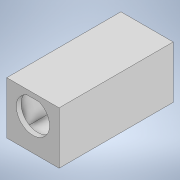
# Autodesk Inventor part: carcasaXeotype_FLEX-SENSOR
Saved by Autodesk Inventor 2020 (Build 240168000, 168)
## iProperties
Created: 2021-04-10
Part Number: carcasaXeotype_FLEX-SENSOR
Material: Generic
Document SubType Name: Modeling
Designer: Vlasciar
Density: 1 g/cm^3
Appearance: Default
Author: Vlasciar
Autodesk Inventor part; units mm, degrees
ref_plane "YZ Plane" through (0, 0, 0) normal (1, 0, 0) x (0, 1, 0)
ref_plane "XZ Plane" through (0, 0, 0) normal (0, 1, 0) x (-1, 0, 0)
ref_plane "XY Plane" through (0, 0, 0) normal (0, 0, 1) x (1, 0, 0)
sketch "Sketch1" plane through (0, 0, 0) normal (0, 1, 0) x (-1, 0, 0)
  line L0 (-5.5, -12) -> (5.5, -12)
  line L1 (5.5, -12) -> (5.5, 12)
  line L2 (5.5, 12) -> (-5.5, 12)
  line L3 (-5.5, 12) -> (-5.5, -12)
  line L4 (-5.5, -12) -> (5.5, 12) construction
  line L5 (5.5, -12) -> (-5.5, 12) construction
  point P0 (0, 0)
  dimension "d0" = 11
  dimension "d1" = 24
  constraints: 12 end point, 2 midpoint, 2 parallel, 1 horizontal, 1 perpendicular
  measures "d0" distance of L1.end L2.end
  measures "d1" distance of L0.end L1.end
extrude "Extrusion1" add sketch "Sketch1" along normal blind 10
shell "Shell1" thickness 1 removed faces 1 at (1.8333, 10, 4)
sketch "Sketch2" plane through (-5.5, 0, 12) normal (0, 0, 1) x (1, 0, 0)
  line L0 (0, 10) -> (11, 10) projected
  circle A0 centre (5.5, 6.75) radius 3.5
  point P0 (5.5, 0)
  point P1 (4.201, 10)
  point P2 (6.799, 10)
  dimension "d5" = 7
  dimension "d6" = 0.25
  constraints: 1 centre point
  measures "d5" diameter of A0
  measures "d6" distance edge to line of A0 L0
extrude "Extrusion2" cut sketch "Sketch2" against normal blind 9 contours L0 A0 picked at (4.7002, 5.9949)
sketch "Sketch3" plane through (0, 10, 0) normal (0, 1, 0) x (1, 0, 0)
  line L0 (1.299, -12) -> (5.5, -12) projected
  line L1 (5.5, -12) -> (5.5, 12) projected
  line L2 (5.5, 12) -> (-5.5, 12) projected
  line L3 (-5.5, 12) -> (-5.5, -12) projected
  line L4 (-5.5, -12) -> (-1.299, -12) projected
  line L5 (-5.5, 12) -> (5.5, 12)
  line L6 (5.5, 12) -> (5.5, -12)
  line L7 (5.5, -12) -> (-5.5, -12)
  line L8 (-5.5, -12) -> (-5.5, 12)
  point P0 (0, 0)
  point P1 (-1.299, -12)
  constraints: 8 end point, 2 parallel, 1 horizontal, 1 perpendicular
extrude "Extrusion3" add sketch "Sketch3" along normal blind 1
sketch "Sketch5" plane through (0, 0, 0) normal (0, -1, 0) x (1, 0, 0)
  line L0 (4.5, -11) -> (-4.5, -11) projected
  line L1 (3, -11) -> (-3, -11)
  line L2 (-3, -11) -> (-3, -6.5)
  line L3 (-2.25, -5.75) -> (2.25, -5.75)
  line L4 (3, -6.5) -> (3, -11)
  arc A0 (3, -6.5) -> (2.25, -5.75) centre (2.25, -6.5) ccw
  arc A1 (-2.25, -5.75) -> (-3, -6.5) centre (-2.25, -6.5) ccw
  line L5 (-5.5, -12) -> (-5.5, 12) projected
  line L6 (5.5, 12) -> (5.5, -12) projected
  line L7 (-3, -11) -> (-5.5, -11)
  line L8 (3, -11) -> (5.5, -11)
  point P0 (0, 0)
  point P1 (3, -5.75)
  dimension "d19" = 5.25
  dimension "d20" = 0.75
  dimension "d23" = 6
  constraints: 12 end point, 7 point on line, 4 point on circle, 4 tangent, 2 centre point, 2 parallel, 1 collinear, 1 equal radius, 1 horizontal, 1 perpendicular
  measures "d19" distance of point (3, -5.75) L1.start
  measures "d20" radius of A0
  measures "d23" distance between parallel lines of L2 L4
extrude "Extrusion5" cut sketch "Sketch5" against normal blind 10
body "Solid1"
